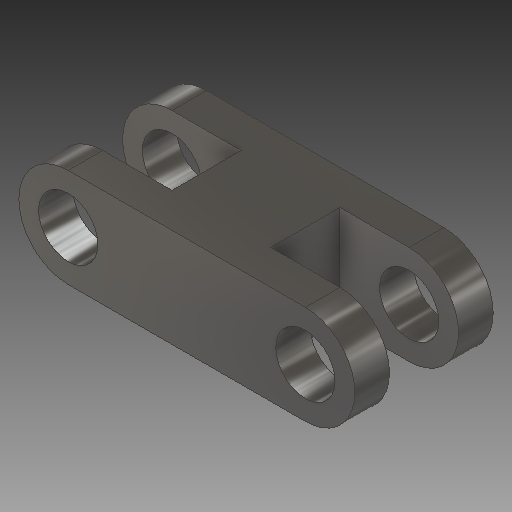
# Autodesk Inventor part: ConnectBoard
Saved by Autodesk Inventor 2019 (Build 230136000, 136)
## iProperties
Created: 2018-12-28
Part Number: ConnectBoard
Material: 钢，高强度，低合金
Document SubType Name: Modeling
Designer: JianQiao Hu
Density: 7.85 g/cm^3
Appearance: 钢 - 抛光
Author: JianQiao Hu
Autodesk Inventor part; units mm, degrees
ref_plane "YZ Plane" through (0, 0, 0) normal (1, 0, 0) x (0, 1, 0)
ref_plane "XZ Plane" through (0, 0, 0) normal (0, 1, 0) x (-1, 0, 0)
ref_plane "XY Plane" through (0, 0, 0) normal (0, 0, 1) x (1, 0, 0)
sketch "草图1" plane through (0, 0, 0) normal (0, 0, 1) x (1, 0, 0)
  line L0 (-44.0519, -22.2048) -> (24.7481, -22.2048)
  line L1 (-44.0519, -22.2048) -> (-44.0519, 41.5952)
  line L2 (-104.0519, 2.7952) -> (15.9481, 2.7952)
  line L3 (15.9481, -47.2048) -> (-104.0519, -47.2048)
  line L4 (-104.0519, 2.7952) -> (15.9481, -47.2048) construction
  line L5 (15.9481, 2.7952) -> (-104.0519, -47.2048) construction
  arc A0 (15.9481, -47.2048) -> (15.9481, 2.7952) centre (15.9481, -22.2048) ccw
  arc A1 (-104.0519, 2.7952) -> (-104.0519, -47.2048) centre (-104.0519, -22.2048) ccw
  circle A2 centre (-104.0519, -22.2048) radius 15
  circle A3 centre (15.9481, -22.2048) radius 15
  dimension "d2" = 25
  dimension "d3" = 50
  dimension "d4" = 120
  dimension "d7" = 30
  dimension "d8" = 30
  dimension "d14" = 50
  constraints: 12 end point, 4 centre point, 4 point on circle, 2 coincident, 2 horizontal, 2 midpoint, 2 point on line, 1 parallel, 1 vertical
  measures "d2" radius of A0
  measures "d3" diameter of A1
  measures "d4" distance of A0.centre A1.centre
  measures "d7" diameter of A2
  measures "d8" diameter of A3
  measures "d14" distance between parallel lines of L2 L3
extrude "拉伸1" add sketch "草图1" along normal blind 70
sketch "草图2" plane through (-104.0519, 2.7952, 0) normal (0, 1, 0) x (1, 0, 0)
  line L0 (0, 0) -> (120, 0) projected
  line L1 (60, 0) -> (60, -70)
  line L2 (120, -70) -> (0, -70) projected
  line L3 (-25, 0) -> (-25, -70) projected
  line L4 (-25, -35) -> (145, -35)
  line L5 (145, 0) -> (145, -70) projected
  line L6 (145, -17.5) -> (145, -52.5)
  line L7 (-25, -52.5) -> (-25, -17.5)
  line L8 (-25, -17.5) -> (145, -52.5) construction
  line L9 (145, -17.5) -> (-25, -52.5) construction
  line L10 (35, -17.5) -> (35, -52.5)
  line L11 (85, -17.5) -> (85, -52.5)
  line L12 (145, -52.5) -> (85, -52.5)
  line L13 (35, -52.5) -> (-25, -52.5)
  line L14 (-25, -17.5) -> (35, -17.5)
  line L15 (85, -17.5) -> (145, -17.5)
  point P0 (104.0519, 0)
  point P1 (60, -35)
  dimension "d10" = 60
  dimension "d11" = 60
  dimension "d15" = 35
  dimension "d16" = 17.5
  dimension "d17" = 35
  constraints: 24 end point, 7 midpoint, 6 perpendicular, 5 parallel, 2 horizontal, 1 point on line
  measures "d10" distance between parallel lines of L5 L11
  measures "d11" distance between parallel lines of L3 L10
  measures "d15" distance of L7.start L7.end
  measures "d16" distance between parallel lines of L4 L14
  measures "d17" distance between parallel lines of L15 L12
extrude "拉伸2" cut sketch "草图2" against normal blind 70
